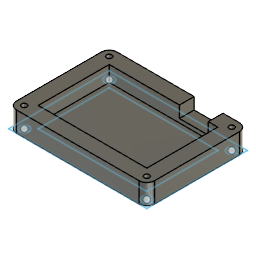
Speedrun pad bottom - James - DONE! (Autodesk Fusion 360 design; units mm, degrees)
part number: 2026-01-23-14-46-17-301
Autodesk Fusion 360 part; units mm, degrees
sketch "Sketch1" plane through (0, 0, 0) normal (0, 0, 1) x (1, 0, 0)
  line L0 (-32.7972, 24.5979) -> (36.9278, 24.5979)
  line L1 (36.9278, 24.5979) -> (36.9278, -20.9771)
  line L2 (36.9278, -20.9771) -> (-32.7972, -20.9771)
  line L3 (-32.7972, -20.9771) -> (-32.7972, 24.5979)
  line L4 (-42.2972, 34.0979) -> (46.4278, 34.0979)
  line L5 (46.4278, 34.0979) -> (46.4278, -30.4771)
  line L6 (46.4278, -30.4771) -> (-42.2972, -30.4771)
  line L7 (-42.2972, -30.4771) -> (-42.2972, 34.0979)
  circle A0 centre (-37.2972, 29.0979) radius 1.7
  circle A1 centre (-37.2972, 29.0979) radius 3
  circle A2 centre (41.4278, 29.0979) radius 1.7
  circle A3 centre (41.4278, 29.0979) radius 3
  circle A4 centre (41.4278, -25.4771) radius 1.7
  circle A5 centre (41.4278, -25.4771) radius 3
  circle A6 centre (-37.2972, -25.4771) radius 1.7
  circle A7 centre (-37.2972, -25.4771) radius 3
  dimension "d14" = 6
  dimension "d18" = 6
  dimension "d22" = 6
  constraint horizontal L0
  constraint vertical L1
  constraint horizontal L2
  constraint vertical L3
  constraint horizontal L4
  constraint vertical L5
  constraint horizontal L6
  constraint vertical L7
  constraint concentric A0 A1
  constraint concentric A2 A3
  constraint concentric A4 A5
  constraint concentric A6 A7
  measures "d14" diameter of A3
  measures "d18" diameter of A5
  measures "d22" diameter of A7
extrude "Extrude1" add sketch "Sketch1" along normal blind 9.9 from surface at 3.1 contours A1 | A3 | A5 | A7 makes body 1 at (44.424, 28.9484, 9.7) makes body 2 at (-34.301, -25.6266, 9.7) makes body 3 at (-34.301, 28.9484, 9.7) makes body 4 at (44.424, -25.6266, 9.7)
extrude "Extrude2" add sketch "Sketch1" along normal blind 13 contours L4 L5 L6 L7 bodies 1 2 3 4
extrude "Extrude3" add sketch "Sketch1" along normal blind 3 contours L0 L1 L2 L3 bodies 1
sketch "Sketch2" plane through (0, 0, 13) normal (0, 0, 1) x (-1, 0, 0)
  circle A0 centre (-41.4278, -29.0979) radius 1.7
  circle A1 centre (-41.4278, 25.4771) radius 1.7
  line L0 (-36.9278, 20.9771) -> (32.7972, 20.9771)
  line L1 (32.7972, 20.9771) -> (32.7972, -24.5979)
  line L2 (32.7972, -24.5979) -> (-36.9278, -24.5979)
  line L3 (-36.9278, -24.5979) -> (-36.9278, 20.9771)
  line L4 (42.2972, 30.4771) -> (-46.4278, 30.4771)
  line L5 (-46.4278, 30.4771) -> (-46.4278, -34.0979)
  line L6 (-46.4278, -34.0979) -> (42.2972, -34.0979)
  line L7 (42.2972, -34.0979) -> (42.2972, 30.4771)
  circle A2 centre (37.2972, 25.4771) radius 1.7
  circle A3 centre (37.2972, -29.0979) radius 1.7
  line L8 (-12.3028, -34.0979) -> (-30.8028, -34.0979)
  line L9 (-30.8028, -34.0979) -> (-30.8028, -24.5979)
  line L10 (-30.8028, -24.5979) -> (-12.3028, -24.5979)
  line L11 (-12.3028, -24.5979) -> (-12.3028, -34.0979)
  line L12 (42.2972, 30.4771) -> (42.2972, -34.0979)
  dimension "d30" = 18.5
  dimension "d31" = 54.6
  constraint horizontal L8
  constraint vertical L9
  constraint horizontal L10
  constraint vertical L11
  constraint coincident L2 L9.end
  constraint coincident L6 L8.start
  measures "d30" distance of L9 L11
  measures "d31" distance of L11 L12
extrude "Extrude4" cut sketch "Sketch2" against normal blind 7.5 contours L2 L6 L8 L9 L10 L11 bodies 1
fillet "Fillet1" radius 5 4 edges at (-42.2972, -30.4771, 6.5) (-42.2972, 34.0979, 6.5) (46.4278, -30.4771, 6.5) (46.4278, 34.0979, 6.5) on bodies 1
